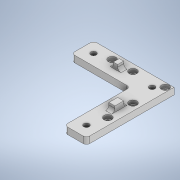
# Autodesk Inventor part: perehodnik
Saved by Autodesk Inventor 2021 (Build 250183000, 183)
## iProperties
Created: 2023-02-16
Part Number: perehodnik
Material: Типовые
Document SubType Name: Modeling
Designer: ignat
Density: 1 g/cm^3
Appearance: По умолчанию
Author: ignat
Autodesk Inventor part; units mm, degrees
ref_plane "YZ Plane" through (0, 0, 0) normal (1, 0, 0) x (0, 1, 0)
ref_plane "XZ Plane" through (0, 0, 0) normal (0, 1, 0) x (-1, 0, 0)
ref_plane "XY Plane" through (0, 0, 0) normal (0, 0, 1) x (1, 0, 0)
sketch "Эскиз1" plane through (0, 0, 0) normal (0, 1, 0) x (-1, 0, 0)
  line L0 (0, 0) -> (0, 80)
  line L1 (0, 80) -> (20, 80)
  line L2 (20, 80) -> (20, 20)
  line L3 (20, 20) -> (73.5, 20)
  line L4 (73.5, 20) -> (73.5, 0)
  line L5 (73.5, 0) -> (0, 0)
  dimension "d0" = 80
  dimension "d1" = 20
  dimension "d2" = 60
  dimension "d3" = 53.5
  constraints: 12 end point, 5 perpendicular, 1 vertical
  measures "d0" distance of L0.start L0.end
  measures "d1" distance of L0.end L1.end
  measures "d2" distance of L1.end L2.end
  measures "d3" distance of L2.end L3.end
extrude "Выдавливание1" add sketch "Эскиз1" along normal blind 6
fillet "Сопряжение1" radius 3 5 edges at (-73.5, 3, 20) (-73.5, 3, 0) (-20, 3, 80) (0, 3, 80) (-20, 3, 20)
sketch "Эскиз2" plane through (0, 6, 0) normal (0, 1, 0) x (1, 0, 0)
  circle A0 centre (-6.25, -31.25) radius 1.75
  circle A1 centre (-4, -4) radius 1.75
  circle A2 centre (-31.25, -6.25) radius 1.75
  circle A3 centre (-50.25, -6.25) radius 1.75
  circle A4 centre (-6.25, -54.25) radius 1.75
  circle A5 centre (-6.25, -54.25) radius 3.5
  circle A6 centre (-6.25, -31.25) radius 3.5
  circle A7 centre (-4, -4) radius 3.5
  circle A8 centre (-31.25, -6.25) radius 3.5
  circle A9 centre (-50.25, -6.25) radius 3.5
  dimension "d7" = 7
  dimension "d8" = 7
  dimension "d9" = 7
  dimension "d10" = 7
  dimension "d11" = 7
  constraints: 15 centre point, 5 coincident
  measures "d7" diameter of A5
  measures "d8" diameter of A6
  measures "d9" diameter of A7
  measures "d10" diameter of A8
  measures "d11" diameter of A9
extrude "Выдавливание2" cut sketch "Эскиз2" against normal through all contours A0 | A1 | A2 | A3 | A4
extrude "Выдавливание3" cut sketch "Эскиз2" against normal blind 3 contours A0 | A1 | A2 | A3 | A4 | A5 | A6 | A7 | A8 | A9
sketch "Эскиз3" plane through (0, 6, 0) normal (0, 1, 0) x (1, 0, 0)
  line L0 (-20, -85.5935) -> (0, -85.5935)
  line L1 (-7.25, -46.75) -> (-12.75, -46.75)
  line L2 (-12.75, -46.75) -> (-12.75, -38.75)
  line L3 (-12.75, -38.75) -> (-7.25, -38.75)
  line L4 (-7.25, -38.75) -> (-7.25, -46.75)
  line L5 (-7.25, -46.75) -> (-12.75, -38.75) construction
  line L6 (-12.75, -46.75) -> (-7.25, -38.75) construction
  line L7 (0, 0) -> (13.4319, 0) construction
  line L8 (-42.75, -12.75) -> (-38.75, -12.75)
  line L9 (-38.75, -12.75) -> (-38.75, -7.25)
  line L10 (-38.75, -7.25) -> (-42.75, -7.25)
  line L11 (-42.75, -7.25) -> (-42.75, -12.75)
  point P0 (-10, -42.75)
  constraints: 24 end point, 3 horizontal, 2 midpoint, 2 parallel, 1 perpendicular
extrude "Выдавливание4" add sketch "Эскиз3" along normal blind 5
sketch "Эскиз4" plane through (0, 6, 0) normal (0, 1, 0) x (1, 0, 0)
  line L0 (-27.1384, -80) -> (-27.1384, -70)
  line L1 (-80, 9.988) -> (-53.75, 9.988)
  circle A0 centre (-10, -70) radius 2.5
  line L2 (-73.5, -29.8806) -> (-63.5, -29.8806)
  circle A1 centre (-63.5, -10) radius 2.5
  point P0 (0, 0)
  dimension "d26" = 10
  dimension "d27" = 5
  dimension "d28" = 10
  dimension "d29" = 5
  constraints: 6 end point, 2 centre point, 2 horizontal, 1 vertical
  measures "d26" distance of L0.start L0.end
  measures "d27" diameter of A0
  measures "d28" distance of L2.start L2.end
  measures "d29" diameter of A1
extrude "Выдавливание5" cut sketch "Эскиз4" against normal through all
sketch "Эскиз5" plane through (0, 0, 0) normal (0, -1, 0) x (1, 0, 0)
  line L0 (0, 77) -> (0, 0) projected
  line L1 (0, 0) -> (-10, 0)
  line L2 (-10, 0) -> (-10, 10)
  line L3 (-10, 10) -> (0, 10)
  line L4 (0, 10) -> (0, 0)
  circle A0 centre (-10, 10) radius 2.5
  circle A1 centre (-10, 10) radius 6
  dimension "d32" = 10
  dimension "d33" = 10
  dimension "d34" = 5
  dimension "d35" = 12
  constraints: 8 end point, 2 centre point, 2 coincident, 2 parallel, 1 horizontal, 1 perpendicular
  measures "d32" distance of L2.end L3.end
  measures "d33" distance of L1.end L2.end
  measures "d34" diameter of A0
  measures "d35" diameter of A1
extrude "Выдавливание6" cut sketch "Эскиз5" against normal through all contours A0 L2 L3 | L3 L2 A0
extrude "Выдавливание7" cut sketch "Эскиз5" against normal blind 3 contours A1 L2 A0 L3 | L3 A0 L2 A1 | A0 L2 L3 | L3 L2 A0
fillet "Сопряжение2" radius 3 4 edges at (-42.75, 6, 10) (-38.75, 6, 10) (-10, 6, 38.75) (-10, 6, 46.75)
